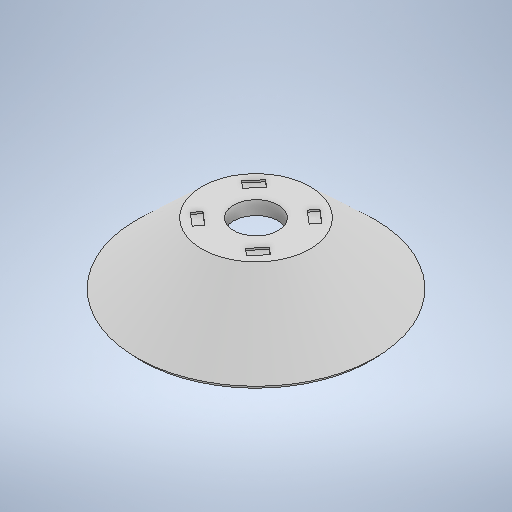
# Autodesk Inventor part: Back Cover
Saved by Autodesk Inventor 2026.2 (Build 302298000, 298)
## iProperties
Created: 2026-01-18
Part Number: Back Cover
Material: Generic
Document SubType Name: Modeling
Designer: daryu
Density: 1 g/cm^3
Appearance: Default
Author: daryu
Autodesk Inventor part; units mm, degrees
ref_plane "YZ Plane" through (0, 0, 0) normal (1, 0, 0) x (0, 1, 0)
ref_plane "XZ Plane" through (0, 0, 0) normal (0, 1, 0) x (-1, 0, 0)
ref_plane "XY Plane" through (0, 0, 0) normal (0, 0, 1) x (1, 0, 0)
sketch "Sketch1" plane through (0, 0, 0) normal (1, 0, 0) x (0, 1, 0)
  line L0 (9.0511, -31.5552) -> (23.3, -16.54)
  line L1 (23.3, -16.54) -> (23.3033, -19.3531)
  line L2 (10.3088, -33.0443) -> (23.3033, -19.3531)
  arc A0 (9.0511, -31.5552) -> (10.3088, -33.0443) centre (56.5754, 7.3116) ccw
  line L3 (9.674, -32.3047) -> (23.3017, -17.9466)
  line L4 (0, 0) -> (23.3, 0)
  line L5 (0, 0) -> (25.6397, 0)
  line L6 (23.3, 0) -> (23.3, -16.54)
  line L7 (23.3, -16.54) -> (15.899, -24.339)
  line L8 (23.3033, -19.3531) -> (25.6397, -16.8915)
  line L9 (23.3, 0) -> (24.3897, 0)
  line L10 (24.3897, 0) -> (24.3897, -16.8)
  line L11 (23.3017, -17.9466) -> (24.3897, -16.8)
  line L12 (25.6397, 0) -> (25.6397, -16.8915)
  line L13 (25.6397, 0) -> (28.254, 0)
  line L14 (28.254, 0) -> (28.254, -15.1793)
  line L15 (28.254, -15.1793) -> (10.9078, -33.6064)
  arc A1 (10.3088, -33.0443) -> (10.9078, -33.6064) centre (31.8453, -10.6914) ccw
  arc A2 (9.674, -32.3047) -> (10.9976, -33.511) centre (15.0193, -27.7689) ccw
  dimension "d0" = 23.3
  dimension "d1" = 16.54
  dimension "d2" = 18.8761
  dimension "d3" = 20.7
  dimension "d4" = 61.3938
  dimension "d5" = 2.8131
  dimension "d6" = 136.5
  dimension "d18" = 16.8
  dimension "d19" = 1.25
  dimension "d22" = 0.9746
  dimension "d25" = 1.9491
  constraints: 32 end point, 7 point on circle, 4 vertical, 3 centre point, 3 horizontal, 2 collinear, 2 parallel, 2 point on line, 1 midpoint
  measures "d0" distance of L4.start L4.end
  measures "d1" distance of L4.end L0.end
  measures "d2" distance of L2.start L1.end
  measures "d3" distance of L0.end L0.start
  measures "d4" radius of A0
  measures "d5" distance of L0.end L1.end
  measures "d6" angle of L7 L6
  measures "d18" distance of L9.end L10.end
  measures "d19" distance of L9.end L5.end
  measures "d22" distance of L2.start L3.start
  measures "d25" distance of L2.start L0.start
revolve "Revolution1" add sketch "Sketch1" angle 360 about axis through (0, 0, 0) along (0, 1, 0) contours L3 L1 L2 A2 | L11 L10 L5 L12 L8 L1 | L2 L8 L12 L13 L14 L15 A2
sketch "Sketch3" plane through (0, 28.254, 0) normal (0, 1, 0) x (1, 0, 0)
  point P0 (0, 0)
hole "Hole2" at (0, 28.254, 0) direction (0, -1, 0) diameter 12.5 end through all
sketch "Sketch4" plane through (0, 28.254, 0) normal (0, 1, 0) x (1, 0, 0)
  line L0 (-5.9666, 8.9326) -> (-7.9148, 10.5784)
  line L1 (-7.9148, 10.5784) -> (-10.9871, 6.9417)
  line L2 (-10.9871, 6.9417) -> (-9.0388, 5.2958)
  line L3 (-9.0388, 5.2958) -> (-5.9666, 8.9326)
  line L4 (-6.9417, -10.9871) -> (-5.2958, -9.0388)
  line L5 (-8.9326, -5.9666) -> (-10.5784, -7.9148)
  line L6 (-10.5784, -7.9148) -> (-6.9417, -10.9871)
  line L7 (-5.2958, -9.0388) -> (-8.9326, -5.9666)
  line L8 (10.9871, -6.9417) -> (9.0388, -5.2958)
  line L9 (5.9666, -8.9326) -> (7.9148, -10.5784)
  line L10 (7.9148, -10.5784) -> (10.9871, -6.9417)
  line L11 (9.0388, -5.2958) -> (5.9666, -8.9326)
  line L12 (6.9417, 10.9871) -> (5.2958, 9.0388)
  line L13 (8.9326, 5.9666) -> (10.5784, 7.9148)
  line L14 (10.5784, 7.9148) -> (6.9417, 10.9871)
  line L15 (5.2958, 9.0388) -> (8.9326, 5.9666)
  point P0 (0, 0)
  point P1 (-10.0129, 6.1188)
  point P2 (-6.1188, -10.0129)
  point P3 (10.0129, -6.1188)
  point P4 (6.1188, 10.0129)
  dimension "d33" = 4.7607
  dimension "d34" = 2.5504
  dimension "d35" = 5.2958
  dimension "d36" = 9.0388
  dimension "d37" = 6.1188
  dimension "d40" = 360
  constraints: 32 end point, 2 parallel, 1 midpoint, 1 perpendicular, 37 other
  measures "d33" distance of L2.end L0.start
  measures "d34" distance of L0.start L0.end
  measures "d35" vertical distance of point (0, 0) L2.end
  measures "d36" horizontal distance of point (0, 0) L2.end
  measures "d37" vertical distance of point (0, 0) point (-10.013, 6.119)
extrude "Extrusion1" cut sketch "Sketch4" against normal blind 0.5
body "Solid1"
